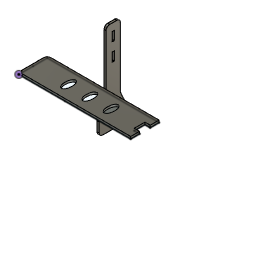
Sweeper v7 (Autodesk Fusion 360 design; units mm, degrees)
Autodesk Fusion 360 part; units mm, degrees
note: some values were not read from the file. Set by a fixed rule: which sketch regions a step uses.
sketch "Sketch1" plane through (0, 0, 0) normal (0, 0, 1) x (1, 0, 0)
  line L0 (65, 0) -> (157.5, 0)
  line L1 (157.5, 0) -> (157.5, 12.5)
  line L2 (157.5, 12.5) -> (150, 12.5)
  line L3 (150, 12.5) -> (150, 27.5)
  line L4 (150, 27.5) -> (157.5, 27.5)
  line L5 (157.5, 27.5) -> (157.5, 40)
  line L6 (157.5, 40) -> (0, 40)
  line L7 (0, 40) -> (0, 20)
  line L8 (0, 20) -> (0, 0)
  line L9 (0, 0) -> (65, 0)
  dimension "d1" = 157.5
  dimension "d2" = 12.5
  dimension "d3" = 7.5
  dimension "d4" = 15
  dimension "d5" = 7.5
  dimension "d6" = 12.5
  constraint horizontal L0
  constraint perpendicular L0 L1
  constraint perpendicular L1 L2
  constraint perpendicular L2 L3
  constraint perpendicular L3 L4
  constraint perpendicular L4 L5
  constraint perpendicular L5 L6
  constraint perpendicular L6 L7
  constraint coincident L8.end L9.start
  constraint parallel L7 L8
  constraint perpendicular L8 L9
  measures "d1" distance of L8.end L0.end
  measures "d2" distance of L0.end L1.end
  measures "d3" distance of L1.end L2.end
  measures "d4" distance of L2.end L3.end
  measures "d5" distance of L3.end L4.end
  measures "d6" distance of L4.end L5.end
extrude "Extrude1" add sketch "Sketch1" along normal blind 3 makes body 1
copy_body "Body->Comp1" bodies 1 removing the originals makes body 2 in component "Component"
sketch "Sketch3" plane through (0, 0, 0) normal (1, 0, 0) x (0, 1, 0)
  line L0 (150, 0) -> (110, 0)
  line L1 (110, 0) -> (110, -130)
  line L2 (110, -130) -> (150, -130)
  line L3 (150, -130) -> (150, 0)
  line L4 (131.6139, -10.4979) -> (128.6139, -10.4979)
  line L5 (128.6139, -10.4979) -> (128.6139, -22.9979)
  line L6 (128.6139, -22.9979) -> (131.6139, -22.9979)
  line L7 (131.6139, -22.9979) -> (131.6139, -10.4979)
  line L8 (128.6139, -35.4979) -> (128.6139, -47.9979)
  line L9 (128.6139, -47.9979) -> (131.6139, -47.9979)
  line L10 (131.6139, -47.9979) -> (131.6139, -35.4979)
  line L11 (131.6139, -35.4979) -> (128.6139, -35.4979)
  arc A0 (120, 0) -> (120, -90) centre (5, -45) ccw
  line L12 (120, 0) -> (120, -90)
  arc A1 (140, -90) -> (140, 0) centre (255, -45) ccw
  line L13 (140, 0) -> (140, -90)
  dimension "d9" = 40
  dimension "d10" = 130
  dimension "d11" = 3
  dimension "d12" = 12.5
  dimension "d15" = 0
  dimension "d16" = -25
  constraint horizontal L0
  constraint vertical L1
  constraint horizontal L2
  constraint vertical L3
  constraint horizontal L4
  constraint vertical L5
  constraint horizontal L6
  constraint vertical L7
  constraint coincident L0 A0.start
  constraint perpendicular L0 L12
  constraint coincident L0 A1.end
  constraint perpendicular L0 L13
  measures "d9" distance of L0.start L0.end
  measures "d10" distance of L0.start L2.end
  measures "d11" distance of L4.start L4.end
  measures "d12" distance of L4.start L6.end
extrude "Extrude3" add sketch "Sketch3" along normal blind 3 separate body contours L0 L1 L2 L3 A0 L12 A1 L13 makes body 3
copy_body "Body->Comp2" bodies 3 removing the originals makes body 4 in component "Component'"
sketch "Sketch4" plane through (0, 0, 3) normal (0, 0, 1) x (-1, 0, 0)
  line L0 (0, 0) -> (-157.5, 0)
  line L1 (-157.5, 0) -> (-157.5, -12.5)
  line L2 (-157.5, -12.5) -> (-150, -12.5)
  line L3 (-150, -12.5) -> (-150, -27.5)
  line L4 (-150, -27.5) -> (-157.5, -27.5)
  line L5 (-157.5, -27.5) -> (-157.5, -40)
  line L6 (-157.5, -40) -> (0, -40)
  line L7 (0, -40) -> (0, 0)
  ellipse E0 centre (-50, -20) end of major axis (-50, -30) minor radius 5
  line L8 (-50, -10) -> (-50, -30)
  line L9 (-55, -20) -> (-45, -20)
  ellipse E1 centre (-80, -20) end of major axis (-80, -30) minor radius 5
  ellipse E2 centre (-110, -20) end of major axis (-110, -30) minor radius 5
  dimension "d21" = 10
  dimension "d24" = -60
  dimension "d25" = 0
  constraint vertical L8
  constraint coincident E0 L8.start
  constraint coincident E0 L8.end
  constraint coincident E0 L9.start
  constraint coincident E0 L9.end
  measures "d21" distance of E0
extrude "Extrude1'" cut sketch "Sketch4" against normal blind 10 contours E0 L8 L9 | E0 L8 L9 | E0 L8 L9 | E0 L8 L9 | E1 | E2 bodies 2 in component "Component"
fillet "Fillet1" radius 5 8 edges at (1.5, 120, 0) (1.5, 140, 0) (1.5, 140, -90) (1.5, 150, -110) (1.5, 150, -130) (1.5, 120, -90) (1.5, 110, -110) (1.5, 110, -130) on bodies 4 in component "Component'"
fillet "Fillet1'" radius 5 2 edges at (0, 40, 1.5) (0, 0, 1.5) on bodies 2 in component "Component"
component "Component" placed x (1, 0, 0) y (0, 1, 0) z (0, 0, 1) at (0, 0, 0)
component "Component'" placed x (1, 0, 0) y (0, 1, 0) z (0, 0, 1) at (0, 0, 0)
